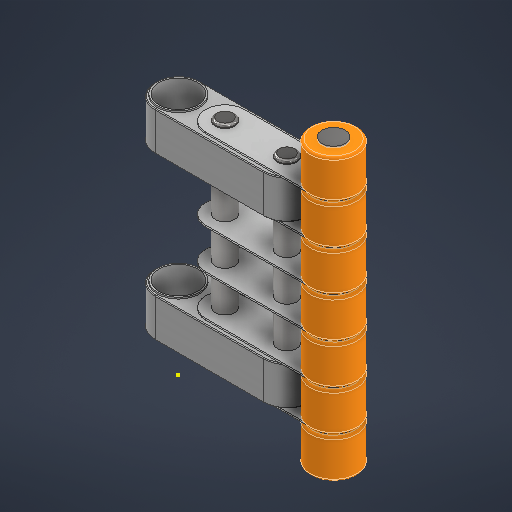
# Autodesk Inventor part: TILES GRIP ROLLERS
Saved by Autodesk Inventor 2025 (Build 290162000, 162)
## iProperties
Created: 2024-05-27
Part Number: TILES GRIP ROLLERS
Material: Generic
Document SubType Name: Modeling
Designer: zulet
Density: 1 g/cm^3
Appearance: Default
Author: zulet
Autodesk Inventor part; units mm, degrees
ref_plane "YZ Plane" through (0, 0, 0) normal (1, 0, 0) x (0, 1, 0)
ref_plane "XZ Plane" through (0, 0, 0) normal (0, 1, 0) x (-1, 0, 0)
sketch "Sketch1" plane through (0, 0, 0) normal (0, 1, 0) x (-1, 0, 0)
  circle A0 centre (0, 0) radius 25
  circle A1 centre (-60, 0) radius 12.5
  circle A2 centre (-140, 0) radius 12.5
  circle A3 centre (-200, 0) radius 15
  line L0 (0, 0) -> (-200, 0) construction
  line L1 (-60, 0) -> (-200, 0) construction
  line L2 (-60, 25) -> (-200, 25)
  line L3 (-200, -25) -> (-60, -25)
  arc A4 (-60, -25) -> (-60, 25) centre (-60, 0) ccw
  arc A5 (-200, 25) -> (-200, -25) centre (-200, 0) ccw
  point P0 (-130, 0)
  dimension "d0" = 50
  dimension "d1" = 25
  dimension "d2" = 25
  dimension "d3" = 30
  dimension "d4" = 200
  dimension "d5" = 140
  dimension "d6" = 60
  dimension "d7" = 50
  constraints: 10 end point, 6 centre point, 4 point on circle, 4 tangent, 2 point on line, 1 coincident, 1 collinear, 1 horizontal, 1 midpoint, 1 parallel
  measures "d0" diameter of A0
  measures "d1" diameter of A1
  measures "d2" diameter of A2
  measures "d3" diameter of A3
  measures "d4" distance of L0.start L0.end
  measures "d5" distance of point (0, 0) A2.centre
  measures "d6" distance of point (0, 0) L1.start
  measures "d7" diameter of A5
extrude "Extrusion1" add sketch "Sketch1" along normal blind 262 contours A1 | A2 | A3
extrude "Extrusion2" add sketch "Sketch1" along normal blind 2 separate body contours A4 L3 A5 L2
sketch "Sketch2" plane through (0, 2, 0) normal (0, 1, 0) x (1, 0, 0)
  circle A0 centre (0, 0) radius 25 projected
  circle A1 centre (60, 0) radius 12.5 projected
  circle A2 centre (140, 0) radius 12.5 projected
  line L0 (0, 0) -> (140, 0) construction
  line L1 (0, -30) -> (140, -30)
  line L2 (140, 30) -> (0, 30)
  arc A3 (0, 30) -> (0, -30) centre (0, 0) ccw
  arc A4 (140, -30) -> (140, 30) centre (140, 0) ccw
  point P0 (70, 0)
  dimension "d12" = 60
  constraints: 8 end point, 4 point on circle, 4 tangent, 2 centre point, 1 horizontal, 1 midpoint, 1 parallel
  measures "d12" diameter of A4
extrude "Extrusion3" add sketch "Sketch2" along normal blind 50 separate body
sketch "Sketch3" plane through (0, 52, 0) normal (0, 1, 0) x (1, 0, 0)
  circle A0 centre (0, 0) radius 27
  circle A1 centre (0, 0) radius 25 projected
  dimension "d15" = 2
  constraints: 1 centre point, 1 coincident
  measures "d15" radial gap between concentric circles of A1 A0
extrude "Extrusion4" add sketch "Sketch3" along normal blind 2 and the other way blind 52 bodies 3
fillet "Fillet1" radius 1 8 edges at (170, 52, 0) (70, 52, -30) (-30, 52, 0) (70, 52, 30) (170, 2, 0) (70, 2, -30) (-30, 2, 0) (70, 2, 30)
pattern_linear "Rectangular Pattern1" count 6 spacing 52 along (0, 1, 0) bodies 2
pattern_linear "Rectangular Pattern2" count 2 spacing 208 along (0, 1, 0) bodies 3
sketch "Sketch4" plane through (200, 262, 0) normal (0, 1, 0) x (1, 0, 0)
  circle A0 centre (0, 0) radius 15 projected
  circle A1 centre (-60, 0) radius 12.5 projected
  circle A2 centre (-140, 0) radius 12.5 projected
  point P0 (-200, 0)
extrude "Extrusion5" add sketch "Sketch4" along normal blind 52 contours A0 bodies 1
sketch "Sketch5" plane through (200, 0, 0) normal (0, -1, 0) x (1, 0, 0)
  circle A0 centre (0, 0) radius 15 projected
  circle A1 centre (-140, 0) radius 12.5 projected
  circle A2 centre (-60, 0) radius 12.5 projected
  point P0 (-200, 0)
extrude "Extrusion6" add sketch "Sketch5" along normal blind 52 contours A0 bodies 1
extrude "Extrusion7" add sketch "Sketch4" along normal blind 4 contours A1 | A2 bodies 1
extrude "Extrusion8" add sketch "Sketch5" along normal blind 4 contours A1 | A2 bodies 1
fillet "Fillet2" radius 3 4 edges at (47.5, 266, 0) (127.5, 266, 0) (47.5, -4, 0) (127.5, -4, 0)
sketch "Sketch6" plane through (200, -52, 0) normal (0, -1, 0) x (1, 0, 0)
  point P0 (-200, 0)
ref_plane "Work Plane1" through (200, -50, 0) normal (0, -1, 0) x (1, 0, 0)
sketch "Sketch7" plane through (200, -50, 0) normal (0, -1, 0) x (1, 0, 0)
  circle A0 centre (0, 0) radius 15 projected
  circle A1 centre (0, 0) radius 30
  point P0 (-200, 0)
  dimension "d37" = 60
  constraints: 1 centre point, 1 coincident
  measures "d37" diameter of A1
extrude "Extrusion9" add sketch "Sketch7" against normal blind 50 separate body
fillet "Fillet3" radius 3 2 edges at (170, 0, 0) (170, -50, 0)
pattern_linear "Rectangular Pattern3" count 7 spacing 52 along (0, 1, 0) bodies 4
body "Solid1"
body "Solid2"
body "Solid3"
body "Solid4"
